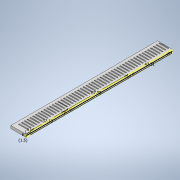
# Autodesk Inventor part: purple reign bridge
Saved by Autodesk Inventor 2022.1 (Build 261234000, 234)
## iProperties
Created: 2023-04-24
Part Number: purple reign bridge
Material: Generic
Document SubType Name: Modeling
Designer: jerald_vanblaricom
Density: 1 g/cm^3
Appearance: Default
Author: jerald_vanblaricom
Autodesk Inventor part; units mm, degrees
ref_plane "YZ Plane" through (0, 0, 0) normal (1, 0, 0) x (0, 1, 0)
ref_plane "XZ Plane" through (0, 0, 0) normal (0, 1, 0) x (-1, 0, 0)
ref_plane "XY Plane" through (0, 0, 0) normal (0, 0, 1) x (1, 0, 0)
sketch "Sketch1" plane through (0, 0, 0) normal (0, 1, 0) x (-1, 0, 0)
  line L0 (-8, 75) -> (8, 75)
  line L1 (8, 75) -> (8, -75)
  line L2 (8, -75) -> (-8, -75)
  line L3 (-8, -75) -> (-8, 75)
  line L4 (-8, 75) -> (8, -75) construction
  line L5 (8, 75) -> (-8, -75) construction
  line L6 (-5, -72) -> (5, -72)
  line L7 (5, -72) -> (5, 72)
  line L8 (5, 72) -> (-5, 72)
  line L9 (-5, 72) -> (-5, -72)
  line L10 (-5, -72) -> (5, 72) construction
  line L11 (5, -72) -> (-5, 72) construction
  point P0 (0, 0)
  dimension "d0" = 16
  dimension "d1" = 150
  dimension "d2" = 10
  dimension "d3" = 144
  dimension "d4" = 3
  constraints: 24 end point, 4 midpoint, 4 parallel, 2 horizontal, 2 perpendicular
  measures "d0" distance of L1.end L2.end
  measures "d1" distance of L0.end L1.end
  measures "d2" distance of L8.end L7.end
  measures "d3" distance of L7.end L6.end
  measures "d4" distance between parallel lines of L0 L8
extrude "Extrusion1" add sketch "Sketch1" along normal blind 3
sketch "Sketch2" plane through (0, 3, 0) normal (0, 1, 0) x (1, 0, 0)
  line L0 (8, 75) -> (-8, 75) projected
  line L1 (-8, 75) -> (-8, -75) projected
  line L2 (-8, -75) -> (8, -75) projected
  line L3 (8, -75) -> (8, 75) projected
  line L4 (5, 72) -> (5, -72) projected
  line L5 (5, -72) -> (-5, -72) projected
  line L6 (-5, -72) -> (-5, 72) projected
  line L7 (-5, 72) -> (5, 72) projected
  line L8 (-5, -72) -> (-5, -70)
  line L9 (-5, -72) -> (-5, 72) projected
  line L10 (-5, -70) -> (5, -70)
  line L11 (5, 72) -> (5, -72) projected
  line L12 (5, -70) -> (5, -72)
  line L13 (5, -72) -> (-5, -72) projected
  line L14 (-5, -72) -> (5, -72)
  line L15 (-5, -68.98) -> (5, -68.98)
  line L16 (-5, -66.98) -> (5, -66.98)
  line L17 (-5, -68.98) -> (-5, -66.98)
  line L18 (5, -66.98) -> (5, -68.98)
  line L19 (-5, -65.96) -> (5, -65.96)
  line L20 (-5, -63.96) -> (5, -63.96)
  line L21 (-5, -65.96) -> (-5, -63.96)
  line L22 (5, -63.96) -> (5, -65.96)
  line L23 (-5, -62.94) -> (5, -62.94)
  line L24 (-5, -60.94) -> (5, -60.94)
  line L25 (-5, -62.94) -> (-5, -60.94)
  line L26 (5, -60.94) -> (5, -62.94)
  line L27 (-5, -59.92) -> (5, -59.92)
  line L28 (-5, -57.92) -> (5, -57.92)
  line L29 (-5, -59.92) -> (-5, -57.92)
  line L30 (5, -57.92) -> (5, -59.92)
  line L31 (-5, -56.9) -> (5, -56.9)
  line L32 (-5, -54.9) -> (5, -54.9)
  line L33 (-5, -56.9) -> (-5, -54.9)
  line L34 (5, -54.9) -> (5, -56.9)
  line L35 (-5, -53.88) -> (5, -53.88)
  line L36 (-5, -51.88) -> (5, -51.88)
  line L37 (-5, -53.88) -> (-5, -51.88)
  line L38 (5, -51.88) -> (5, -53.88)
  line L39 (-5, -50.86) -> (5, -50.86)
  line L40 (-5, -48.86) -> (5, -48.86)
  line L41 (-5, -50.86) -> (-5, -48.86)
  line L42 (5, -48.86) -> (5, -50.86)
  line L43 (-5, -47.84) -> (5, -47.84)
  line L44 (-5, -45.84) -> (5, -45.84)
  line L45 (-5, -47.84) -> (-5, -45.84)
  line L46 (5, -45.84) -> (5, -47.84)
  line L47 (-5, -44.82) -> (5, -44.82)
  line L48 (-5, -42.82) -> (5, -42.82)
  line L49 (-5, -44.82) -> (-5, -42.82)
  line L50 (5, -42.82) -> (5, -44.82)
  line L51 (-5, -41.8) -> (5, -41.8)
  line L52 (-5, -39.8) -> (5, -39.8)
  line L53 (-5, -41.8) -> (-5, -39.8)
  line L54 (5, -39.8) -> (5, -41.8)
  line L55 (-5, -38.78) -> (5, -38.78)
  line L56 (-5, -36.78) -> (5, -36.78)
  line L57 (-5, -38.78) -> (-5, -36.78)
  line L58 (5, -36.78) -> (5, -38.78)
  line L59 (-5, -35.76) -> (5, -35.76)
  line L60 (-5, -33.76) -> (5, -33.76)
  line L61 (-5, -35.76) -> (-5, -33.76)
  line L62 (5, -33.76) -> (5, -35.76)
  line L63 (-5, -32.74) -> (5, -32.74)
  line L64 (-5, -30.74) -> (5, -30.74)
  line L65 (-5, -32.74) -> (-5, -30.74)
  line L66 (5, -30.74) -> (5, -32.74)
  line L67 (-5, -29.72) -> (5, -29.72)
  line L68 (-5, -27.72) -> (5, -27.72)
  line L69 (-5, -29.72) -> (-5, -27.72)
  line L70 (5, -27.72) -> (5, -29.72)
  line L71 (-5, -26.7) -> (5, -26.7)
  line L72 (-5, -24.7) -> (5, -24.7)
  line L73 (-5, -26.7) -> (-5, -24.7)
  line L74 (5, -24.7) -> (5, -26.7)
  line L75 (-5, -23.68) -> (5, -23.68)
  line L76 (-5, -21.68) -> (5, -21.68)
  line L77 (-5, -23.68) -> (-5, -21.68)
  line L78 (5, -21.68) -> (5, -23.68)
  line L79 (-5, -20.66) -> (5, -20.66)
  line L80 (-5, -18.66) -> (5, -18.66)
  line L81 (-5, -20.66) -> (-5, -18.66)
  line L82 (5, -18.66) -> (5, -20.66)
  line L83 (-5, -17.64) -> (5, -17.64)
  line L84 (-5, -15.64) -> (5, -15.64)
  line L85 (-5, -17.64) -> (-5, -15.64)
  line L86 (5, -15.64) -> (5, -17.64)
  line L87 (-5, -14.62) -> (5, -14.62)
  line L88 (-5, -12.62) -> (5, -12.62)
  line L89 (-5, -14.62) -> (-5, -12.62)
  line L90 (5, -12.62) -> (5, -14.62)
  line L91 (-5, -11.6) -> (5, -11.6)
  line L92 (-5, -9.6) -> (5, -9.6)
  line L93 (-5, -11.6) -> (-5, -9.6)
  line L94 (5, -9.6) -> (5, -11.6)
  line L95 (-5, -8.58) -> (5, -8.58)
  line L96 (-5, -6.58) -> (5, -6.58)
  line L97 (-5, -8.58) -> (-5, -6.58)
  line L98 (5, -6.58) -> (5, -8.58)
  line L99 (-5, -5.56) -> (5, -5.56)
  line L100 (-5, -3.56) -> (5, -3.56)
  line L101 (-5, -5.56) -> (-5, -3.56)
  line L102 (5, -3.56) -> (5, -5.56)
  line L103 (-5, -2.54) -> (5, -2.54)
  line L104 (-5, -0.54) -> (5, -0.54)
  line L105 (-5, -2.54) -> (-5, -0.54)
  line L106 (5, -0.54) -> (5, -2.54)
  line L107 (-5, 0.48) -> (5, 0.48)
  line L108 (-5, 2.48) -> (5, 2.48)
  line L109 (-5, 0.48) -> (-5, 2.48)
  line L110 (5, 2.48) -> (5, 0.48)
  line L111 (-5, 3.5) -> (5, 3.5)
  line L112 (-5, 5.5) -> (5, 5.5)
  line L113 (-5, 3.5) -> (-5, 5.5)
  line L114 (5, 5.5) -> (5, 3.5)
  line L115 (-5, 6.52) -> (5, 6.52)
  line L116 (-5, 8.52) -> (5, 8.52)
  line L117 (-5, 6.52) -> (-5, 8.52)
  line L118 (5, 8.52) -> (5, 6.52)
  line L119 (-5, 9.54) -> (5, 9.54)
  line L120 (-5, 11.54) -> (5, 11.54)
  line L121 (-5, 9.54) -> (-5, 11.54)
  line L122 (5, 11.54) -> (5, 9.54)
  line L123 (-5, 12.56) -> (5, 12.56)
  line L124 (-5, 14.56) -> (5, 14.56)
  line L125 (-5, 12.56) -> (-5, 14.56)
  line L126 (5, 14.56) -> (5, 12.56)
  line L127 (-5, 15.58) -> (5, 15.58)
  line L128 (-5, 17.58) -> (5, 17.58)
  line L129 (-5, 15.58) -> (-5, 17.58)
  line L130 (5, 17.58) -> (5, 15.58)
  line L131 (-5, 18.6) -> (5, 18.6)
  line L132 (-5, 20.6) -> (5, 20.6)
  line L133 (-5, 18.6) -> (-5, 20.6)
  line L134 (5, 20.6) -> (5, 18.6)
  line L135 (-5, 21.62) -> (5, 21.62)
  line L136 (-5, 23.62) -> (5, 23.62)
  line L137 (-5, 21.62) -> (-5, 23.62)
  line L138 (5, 23.62) -> (5, 21.62)
  line L139 (-5, 24.64) -> (5, 24.64)
  line L140 (-5, 26.64) -> (5, 26.64)
  line L141 (-5, 24.64) -> (-5, 26.64)
  line L142 (5, 26.64) -> (5, 24.64)
  line L143 (-5, 27.66) -> (5, 27.66)
  line L144 (-5, 29.66) -> (5, 29.66)
  line L145 (-5, 27.66) -> (-5, 29.66)
  line L146 (5, 29.66) -> (5, 27.66)
  line L147 (-5, 30.68) -> (5, 30.68)
  line L148 (-5, 32.68) -> (5, 32.68)
  line L149 (-5, 30.68) -> (-5, 32.68)
  line L150 (5, 32.68) -> (5, 30.68)
  line L151 (-5, 33.7) -> (5, 33.7)
  line L152 (-5, 35.7) -> (5, 35.7)
  line L153 (-5, 33.7) -> (-5, 35.7)
  line L154 (5, 35.7) -> (5, 33.7)
  line L155 (-5, 36.72) -> (5, 36.72)
  line L156 (-5, 38.72) -> (5, 38.72)
  line L157 (-5, 36.72) -> (-5, 38.72)
  line L158 (5, 38.72) -> (5, 36.72)
  line L159 (-5, 39.74) -> (5, 39.74)
  line L160 (-5, 41.74) -> (5, 41.74)
  line L161 (-5, 39.74) -> (-5, 41.74)
  line L162 (5, 41.74) -> (5, 39.74)
  line L163 (-5, 42.76) -> (5, 42.76)
  line L164 (-5, 44.76) -> (5, 44.76)
  line L165 (-5, 42.76) -> (-5, 44.76)
  line L166 (5, 44.76) -> (5, 42.76)
  line L167 (-5, 45.78) -> (5, 45.78)
  line L168 (-5, 47.78) -> (5, 47.78)
  line L169 (-5, 45.78) -> (-5, 47.78)
  line L170 (5, 47.78) -> (5, 45.78)
  line L171 (-5, 48.8) -> (5, 48.8)
  line L172 (-5, 50.8) -> (5, 50.8)
  line L173 (-5, 48.8) -> (-5, 50.8)
  line L174 (5, 50.8) -> (5, 48.8)
  line L175 (-5, 51.82) -> (5, 51.82)
  line L176 (-5, 53.82) -> (5, 53.82)
  line L177 (-5, 51.82) -> (-5, 53.82)
  line L178 (5, 53.82) -> (5, 51.82)
  line L179 (-5, 54.84) -> (5, 54.84)
  line L180 (-5, 56.84) -> (5, 56.84)
  line L181 (-5, 54.84) -> (-5, 56.84)
  line L182 (5, 56.84) -> (5, 54.84)
  line L183 (-5, 57.86) -> (5, 57.86)
  line L184 (-5, 59.86) -> (5, 59.86)
  line L185 (-5, 57.86) -> (-5, 59.86)
  line L186 (5, 59.86) -> (5, 57.86)
  line L187 (-5, 60.88) -> (5, 60.88)
  line L188 (-5, 62.88) -> (5, 62.88)
  line L189 (-5, 60.88) -> (-5, 62.88)
  line L190 (5, 62.88) -> (5, 60.88)
  line L191 (-5, 63.9) -> (5, 63.9)
  line L192 (-5, 65.9) -> (5, 65.9)
  line L193 (-5, 63.9) -> (-5, 65.9)
  line L194 (5, 65.9) -> (5, 63.9)
  line L195 (-5, 66.92) -> (5, 66.92)
  line L196 (-5, 68.92) -> (5, 68.92)
  line L197 (-5, 66.92) -> (-5, 68.92)
  line L198 (5, 68.92) -> (5, 66.92)
  line L199 (-5, 69.94) -> (5, 69.94)
  line L200 (-5, 71.94) -> (5, 71.94)
  line L201 (-5, 69.94) -> (-5, 71.94)
  line L202 (5, 71.94) -> (5, 69.94)
  point P0 (0, 0)
  dimension "d7" = 2
  dimension "d10" = 3.02
  constraints: 384 end point, 188 vertical alignment, 94 collinear, 94 parallel, 2 horizontal, 2 point on line, 1 vertical
  measures "d7" distance of L5.end L8.end
  measures "d10" distance of L5.end L15.start
extrude "Extrusion2" add sketch "Sketch2" against normal blind 3 contours L4 L199 L6 L200 | L4 L195 L6 L196 | L4 L191 L6 L192 | L4 L187 L6 L188 | L4 L183 L6 L184 | L4 L179 L6 L180 | L4 L175 L6 L176 | L4 L171 L6 L172 | L4 L167 L6 L168 | L4 L163 L6 L164 | L4 L159 L6 L160 | L4 L155 L6 L156 | L4 L151 L6 L152 | L4 L147 L6 L148 | L4 L143 L6 L144 | L4 L139 L6 L140 | L4 L135 L6 L136 | L4 L131 L6 L132 | L4 L127 L6 L128 | L4 L123 L6 L124 | L4 L119 L6 L120 | L4 L115 L6 L116 | L4 L111 L6 L112 | L4 L107 L6 L108 | L4 L103 L6 L104 | L4 L99 L6 L100 | L4 L95 L6 L96 | L4 L91 L6 L92 | L4 L87 L6 L88 | L4 L83 L6 L84 | L4 L79 L6 L80 | L4 L75 L6 L76 | L4 L71 L6 L72 | L4 L67 L6 L68 | L4 L63 L6 L64 | L4 L59 L6 L60 | L4 L55 L6 L56 | L4 L51 L6 L52 | L4 L47 L6 L48 | L4 L43 L6 L44 | L4 L39 L6 L40 | L4 L35 L6 L36 | L4 L31 L6 L32 | L4 L27 L6 L28 | L4 L23 L6 L24 | L4 L19 L6 L20 | L4 L15 L6 L16 | L4 L5 L6 L10
sketch "Sketch3" plane through (8, 0, 75) normal (1, 0, 0) x (0, 0, -1)
  line L0 (150, 3) -> (0, 3) projected
  line L1 (0, 3) -> (5, 3)
  line L2 (5, 3) -> (5, 1.5)
  line L3 (150, 0) -> (0, 0) projected
  circle A0 centre (5, 1.5) radius 1
  line L4 (5, 3) -> (42.13, 3)
  line L5 (42.13, 3) -> (42.13, 1.5)
  line L6 (42.13, 3) -> (109.68, 3)
  line L7 (109.68, 3) -> (109.68, 1.5)
  line L8 (0, 3) -> (150, 3) projected
  line L9 (150, 0) -> (150, 3) projected
  line L10 (150, 3) -> (158, 3)
  line L11 (158, 3) -> (158, 0)
  line L12 (158, 0) -> (150, 0)
  line L13 (150, 0) -> (150, 3)
  point P0 (75, 0)
  dimension "d17" = 5
  dimension "d18" = 1.5
  dimension "d19" = 2
  dimension "d20" = 37.13
  dimension "d21" = 1.5
  dimension "d22" = 67.55
  dimension "d23" = 1.5
  dimension "d24" = 8
  constraints: 20 end point, 4 perpendicular, 3 point on line, 2 parallel, 1 centre point, 1 coincident, 1 horizontal
  measures "d17" distance of L0.end L1.end
  measures "d18" distance of L1.end L2.end
  measures "d19" diameter of A0
  measures "d20" distance of L1.end L4.end
  measures "d21" distance of L4.end L5.end
  measures "d22" distance of L4.end L6.end
  measures "d23" distance of L6.end L7.end
  measures "d24" distance of L11.end L12.end
extrude "Extrusion3" add sketch "Sketch3" against normal blind 16 contours L10 L11 L12 L9
sketch "Sketch4" plane through (0, 3, 0) normal (0, 1, 0) x (1, 0, 0)
  line L0 (-5, 71.94) -> (-5, 72) projected
  line L1 (-5, 71.94) -> (5, 71.94)
  line L2 (5, 71.94) -> (5, 72.96)
  line L3 (5, 72.96) -> (-5, 72.96)
  line L4 (-5, 72.96) -> (-5, 71.94)
  line L5 (-5, 75.04) -> (5, 75.04)
  line L6 (5, 76.06) -> (-5, 76.06)
  line L7 (5, 75.04) -> (5, 76.06)
  line L8 (-5, 78.14) -> (5, 78.14)
  line L9 (5, 79.16) -> (-5, 79.16)
  line L10 (5, 78.14) -> (5, 79.16)
  line L11 (-5, 81.24) -> (5, 81.24)
  line L12 (5, 82.26) -> (-5, 82.26)
  line L13 (5, 81.24) -> (5, 82.26)
  line L14 (-5, 82.26) -> (-5, 81.24)
  line L15 (-5, 79.16) -> (-5, 78.14)
  line L16 (-5, 76.06) -> (-5, 75.04)
  point P0 (0, 0)
  dimension "d27" = 10
  dimension "d28" = 1.02
  dimension "d31" = 3.1
  constraints: 32 end point, 4 equal length, 2 vertical, 1 horizontal, 1 perpendicular, 21 other
  measures "d27" distance of L3.end L2.end
  measures "d28" distance of L2.end L1.end
  measures "d31" distance of L0.start L5.start
extrude "Extrusion4" cut sketch "Sketch4" against normal blind 16
sketch "Sketch5" plane through (8, 0, 75) normal (1, 0, 0) x (0, 0, -1)
  line L0 (0, 3) -> (158, 3) projected
  line L1 (0, 3) -> (5, 3)
  line L2 (0, 0) -> (158, 0) projected
  line L3 (0, 0) -> (0, 1.5)
  line L4 (0, 0) -> (0, 3) projected
  line L5 (0, 1.5) -> (158, 1.5)
  line L6 (158, 0) -> (158, 3) projected
  line L7 (5, 0) -> (42.13, 0)
  line L8 (42.13, 0) -> (42.26, 1.5)
  line L9 (42.26, 3) -> (42.26, 0) projected
  line L10 (42.26, 0) -> (109.81, 0)
  line L11 (109.81, 0) -> (109.81, 1.5)
  line L12 (109.81, 0) -> (157.12, 0)
  line L13 (157.12, 0) -> (157.12, 1.5)
  point P0 (75, 0)
  dimension "d38" = 5
  dimension "d39" = 1.5
  dimension "d40" = 37.13
  dimension "d41" = 67.55
  dimension "d42" = 47.31
  constraints: 18 end point, 7 point on line, 3 midpoint, 2 perpendicular
  measures "d38" distance of L0.start L1.end
  measures "d39" distance of L2.start L3.end
  measures "d40" distance of L7.start L7.end
  measures "d41" distance of L9.end L10.end
  measures "d42" distance of L10.end L12.end
sketch "Sketch6" plane through (-8, 0, -83) normal (-1, 0, 0) x (0, 0, 1)
  line L0 (158, 3) -> (0, 3) projected
  line L1 (0, 3) -> (5, 3)
  line L2 (5, 3) -> (42.13, 3)
  line L3 (42.13, 3) -> (109.68, 3)
  line L4 (109.68, 3) -> (156.99, 3)
  circle A0 centre (156.99, 1.5) radius 1
  circle A1 centre (109.68, 1.5) radius 1
  circle A2 centre (42.13, 1.5) radius 1
  circle A3 centre (5, 1.5) radius 1
  point P0 (83, 0)
  dimension "d43" = 5
  dimension "d45" = 37.13
  dimension "d47" = 67.55
  dimension "d49" = 47.31
  dimension "d51" = 2
  dimension "d52" = 2
  dimension "d53" = 2
  dimension "d54" = 2
  constraints: 8 end point, 4 centre point, 4 point on line
  measures "d43" distance of L0.end L1.end
  measures "d45" distance of L1.end L2.end
  measures "d47" distance of L2.end L3.end
  measures "d49" distance of L3.end L4.end
  measures "d51" diameter of A0
  measures "d52" diameter of A1
  measures "d53" diameter of A2
  measures "d54" diameter of A3
extrude "Extrusion5" cut sketch "Sketch6" against normal blind 16
body "Solid1"
